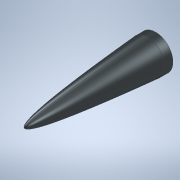
# Autodesk Inventor part: nose
Saved by Autodesk Inventor 2020 (Build 240168000, 168)
## iProperties
Created: 2021-01-23
Part Number: nose
Material: ABS Plastic
Document SubType Name: Modeling
Designer: 0x6f736f646f
Density: 1.06 g/cm^3
Appearance: Iron Gray
Author: 0x6f736f646f
Autodesk Inventor part; units mm, degrees
ref_plane "YZ Plane" through (0, 0, 0) normal (1, 0, 0) x (0, 1, 0)
ref_plane "XZ Plane" through (0, 0, 0) normal (0, 1, 0) x (-1, 0, 0)
ref_plane "XY Plane" through (0, 0, 0) normal (0, 0, 1) x (1, 0, 0)
sketch "Sketch1" plane through (0, 0, 0) normal (1, 0, 0) x (0, 1, 0)
  spline S0 degree 2 poles (16.8, 0.8) (7.4765, 120.8) (0, 120.8) knots 0 0 0 1 1 1
  spline S1 degree 2 poles (15, 0.8) (6.5777, 119) (0, 119) knots 0 0 0 1 1 1
  line L0 (0, 147.71) -> (0, -33.9517) projected
  line L1 (0, 120.8) -> (0, 119)
  line L2 (0.9491, 119) -> (-0.9491, 119) construction
  line L3 (1.0883, 120.8) -> (-1.0883, 120.8) construction
  line L4 (16.8, 0.8) -> (16.8, -7.2)
  line L5 (16.8, -7.2) -> (15.9, -7.2)
  line L6 (15, -3.2) -> (15, 0.8)
  line L7 (15, -3.2) -> (15.9, -3.2)
  line L8 (15.9, -3.2) -> (15.9, -7.2)
  point P0 (0, 118.2679)
  point P1 (0.527, 117.976)
  point P2 (-1.0599, 118.5496)
  point P3 (0, 119.8684)
  point P4 (0.6361, 119.749)
  point P5 (-1.1427, 120.3492)
  dimension "d62" = 15
  dimension "d64" = 118.2
  dimension "d65" = 120
  dimension "d69" = 1.8
  dimension "d70" = 0.9
  dimension "d71" = 0.9
  dimension "d72" = 8
  dimension "d75" = 4
  dimension "d76" = 4
  dimension "d77" = 154.91
  constraints: 16 end point, 4 midpoint, 3 horizontal, 2 perpendicular, 2 point on line, 1 vertical, 13 other
  measures "d62" distance from line of L0 L6.end
  measures "d64" vertical distance of L1.end L6.end
  measures "d65" vertical distance of L1.start L4.start
  measures "d69" distance of L6.end L4.start
  measures "d70" distance between parallel lines of L8 L4
  measures "d71" distance between parallel lines of L6 L8
  measures "d72" distance of L4.start L4.end
  measures "d75" distance of L7.end L5.end
  measures "d76" distance of L6.start L6.end
  measures "d77" distance from line of L0.start L5
revolve "Revolution4" add sketch "Sketch1" angle 360 about axis through (0, 0, 0) along (0, 0, -1)
body "Solid3"
